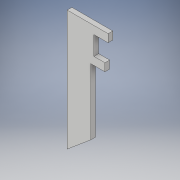
# Autodesk Inventor part: k2_t_side
Saved by Autodesk Inventor 2017 (Build 210142000, 142)
## iProperties
Created: 2017-02-08
Part Number: k2_t_side
Material: Generic
Document SubType Name: Modeling
Designer: herman
Density: 1 g/cm^3
Appearance: Default
Author: herman
Autodesk Inventor part; units mm, degrees
ref_plane "YZ Plane" through (0, 0, 0) normal (1, 0, 0) x (0, 1, 0)
ref_plane "XZ Plane" through (0, 0, 0) normal (0, 1, 0) x (-1, 0, 0)
ref_plane "XY Plane" through (0, 0, 0) normal (0, 0, 1) x (1, 0, 0)
sketch "Sketch2" plane through (0, 0, 0) normal (0, 0, 1) x (1, 0, 0)
  line L0 (-0.8337, 45.419) -> (-0.8337, -31.091)
  line L1 (-0.8337, -31.091) -> (14.1663, -18.5045)
  line L2 (14.1663, -18.5045) -> (14.1663, 23.419)
  line L3 (14.1663, 23.419) -> (23.1663, 23.419)
  line L4 (23.1663, 23.419) -> (23.1663, 28.419)
  line L5 (23.1663, 28.419) -> (16.1663, 28.419)
  line L6 (16.1663, 28.419) -> (16.1663, 40.419)
  line L7 (16.1663, 40.419) -> (25.1663, 40.419)
  line L8 (25.1663, 40.419) -> (25.1663, 45.419)
  line L9 (25.1663, 45.419) -> (-0.8337, 45.419)
  line L10 (16.1663, 28.419) -> (14.1663, 28.419) construction
  line L11 (1.3388, 42.919) -> (15.1663, 42.919)
  line L12 (15.1663, 42.919) -> (15.1663, 41.2824)
  line L13 (15.1663, 41.2824) -> (1.3388, 41.2824)
  line L14 (1.3388, 41.2824) -> (1.3388, 42.919)
  line L15 (11.0785, 23.419) -> (12.1663, 23.419)
  line L16 (12.1663, 23.419) -> (12.1663, -12.6156)
  line L17 (12.1663, -12.6156) -> (11.0785, -12.6156)
  line L18 (11.0785, -12.6156) -> (11.0785, 23.419)
  line L19 (2.2805, -14.4359) -> (12.1663, -14.4359)
  line L20 (12.1663, -14.4359) -> (12.1663, -16.121)
  line L21 (12.1663, -16.121) -> (2.2805, -16.121)
  line L22 (2.2805, -16.121) -> (2.2805, -14.4359)
  dimension "d17" = 2
  dimension "d18" = 7
  dimension "d19" = 9
  dimension "d20" = 5
  dimension "d21" = 5
  dimension "d22" = 15
  dimension "d23" = 12
  dimension "d24" = 2
  dimension "d25" = 46.9235
  dimension "d26" = 130
  constraints: 47 end point, 9 perpendicular, 7 parallel, 5 horizontal, 1 point on line, 1 vertical
  measures "d17" horizontal distance of L2.end L5.end
  measures "d18" distance of L4.end L5.end
  measures "d19" distance of L7.end L6.end
  measures "d20" distance of L3.end L4.end
  measures "d21" distance of L7.end L8.end
  measures "d22" distance between parallel lines of L0 L2
  measures "d23" distance between parallel lines of L5 L7
  measures "d24" distance of L5.end L10.end
  measures "d25" distance of L1.end L10.end
  measures "d26" angle of L1 L2
extrude "Extrusion1" add sketch "Sketch2" along normal blind 3 contours L9 L8 L7 L6 L5 L4 L3 L2 L1 L0 | L11 L12 L13 L14 | L15 L16 L17 L18 | L19 L20 L21 L22
body "Solid2"
